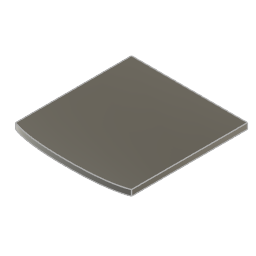
Nebulous Visual (DO NOT USE IN PRINTER) v1 (Autodesk Fusion 360 archive; units mm, degrees)
design "Nebulous Roof"
Autodesk Fusion 360 part; units mm, degrees
sketch "Sketch1" plane through (0, 0, 0) normal (0, 0, 1) x (1, 0, 0)
  line L0 (-100, 100) -> (100, 100)
  line L1 (100, 100) -> (100, -100)
  line L2 (-100, -100) -> (-100, 100)
  spline S0 degree 5 poles (-100, -100) (-98.445, -100.6272) (-95.1746, -101.8432) (-89.7876, -103.5519) (-81.6352, -105.5978) (-69.8139, -107.7572) (-56.3951, -109.5042) (-41.5014, -110.824) (-25.414, -111.707) (-8.5597, -112.1492) (8.5597, -112.1492) (25.414, -111.707) (41.5014, -110.824) (56.3951, -109.5042) (69.8139, -107.7572) (81.6352, -105.5978) (89.7876, -103.5519) (95.1746, -101.8432) (98.445, -100.6272) (100, -100) knots 0 0 0 0 0 0 0.066667 0.133333 0.2 0.266667 0.333333 0.4 0.466667 0.533333 0.6 0.666667 0.733333 0.8 0.866667 0.933333 1 1 1 1 1 1
  point P0 (-50, -110)
  point P1 (50, -110)
  constraint horizontal L0
  constraint vertical L1
  constraint vertical L2
extrude "Extrude1" add sketch "Sketch1" along normal blind 10
